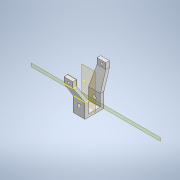
# Autodesk Inventor part: 2020_fixer2
Saved by Autodesk Inventor 2020 (Build 240168000, 168)
## iProperties
Created: 2019-10-23
Part Number: 2020_fixer2
Material: Generic
Document SubType Name: Modeling
Designer: psrob
Density: 1 g/cm^3
Appearance: Default
Author: psrob
Autodesk Inventor part; units mm, degrees
ref_plane "YZ Plane" through (0, 0, 0) normal (1, 0, 0) x (0, 1, 0)
ref_plane "XZ Plane" through (0, 0, 0) normal (0, 1, 0) x (-1, 0, 0)
ref_plane "XY Plane" through (0, 0, 0) normal (0, 0, 1) x (1, 0, 0)
sketch "Sketch1" plane through (0, 0, 0) normal (0, 0, 1) x (1, 0, 0)
  circle A0 centre (-47.5, -10) radius 3 projected
  circle A1 centre (-5, 30) radius 2 projected
  line L0 (-47.5, -10) -> (-2.5, -10)
  line L1 (7.5, 0) -> (-12.5, 0)
  line L2 (-12.5, 0) -> (-12.5, -20)
  line L3 (-12.5, -20) -> (7.5, -20)
  line L4 (7.5, -20) -> (7.5, 0)
  line L5 (7.5, 0) -> (-12.5, -20) construction
  line L6 (-12.5, 0) -> (7.5, -20) construction
  point P0 (0, 0)
  dimension "d0" = 45
  dimension "d1" = 20
  dimension "d2" = 20
  constraints: 14 end point, 2 midpoint, 2 parallel, 2 perpendicular, 1 horizontal
  measures "d0" distance of L0.start L0.end
  measures "d1" distance of L1.start L1.end
  measures "d2" distance of L2.end L1.end
extrude "Extrusion1" add sketch "Sketch1" along normal blind 6 contours L4 L3 L2 L1
ref_plane "Work Plane1" through (0, 0, -20) normal (0, 0, -1) x (-1, 0, 0)
sketch "Sketch2" plane through (0, 0, -20) normal (0, 0, -1) x (-1, 0, 0)
  line L0 (-7.5, -20) -> (-7.5, 0) projected
  line L1 (-7.5, 0) -> (12.5, 0) projected
  line L2 (12.5, 0) -> (12.5, -20) projected
  line L3 (12.5, -20) -> (-7.5, -20) projected
  point P0 (0, 0)
  dimension "d0" = 45
  dimension "d1" = 20
  dimension "d2" = 20
extrude "Extrusion2" add sketch "Sketch2" along normal blind 6
ref_plane "Work Plane2" through (-8, 25, 15) normal (0, 0, 1) x (0, 1, 0)
sketch "Sketch3" plane through (-8, 25, 15) normal (0, 0, 1) x (0, 1, 0)
  circle A0 centre (5, -3) radius 2 projected
  arc A1 (8, -10) -> (10, -8) centre (8, -8) ccw projected
  line L0 (10, -8) -> (10, -3) projected
  line L1 (10, -3) -> (10, 5) projected
  line L2 (0, 5) -> (10, 5) projected
  line L3 (0, 5) -> (0, -3) projected
  line L4 (0, -3) -> (0, -8) projected
  arc A2 (0, -8) -> (2, -10) centre (2, -8) ccw projected
  line L5 (8, -10) -> (2, -10) projected
  circle A3 centre (5, -3) radius 2 projected
  line L6 (0, 4) -> (10, 4)
  line L7 (10, 4) -> (10, -10)
  line L8 (10, -10) -> (0, -10)
  line L9 (0, -10) -> (0, 4)
  line L10 (0, 4) -> (10, -10) construction
  line L11 (10, 4) -> (0, -10) construction
  point P0 (-25, -8)
  point P1 (0, -8)
  point P2 (2, -10)
  point P3 (10, -8)
  dimension "d7" = 10
  dimension "d8" = 14
  constraints: 12 end point, 3 parallel, 2 midpoint, 1 perpendicular
  measures "d7" distance of L6.start L6.end
  measures "d8" distance of L6.end L7.end
extrude "Extrusion3" add sketch "Sketch3" along normal blind 6
sketch "Sketch4" plane through (-13, 25, 15) normal (0, -1, 0) x (1, 0, 0)
  line L0 (0, 0) -> (15, 0) projected
  line L1 (15, 0) -> (15, 6) projected
  line L2 (0, 6) -> (15, 6) projected
  line L3 (0, 0) -> (0, 6) projected
  point P0 (13, -15)
sketch "Sketch5" plane through (-12.5, 0, 0) normal (0, 1, 0) x (1, 0, 0)
  line L0 (20, 0) -> (0, 0) projected
  line L1 (0, 0) -> (0, -6) projected
  line L2 (20, -6) -> (0, -6) projected
  line L3 (20, 0) -> (20, -6) projected
  point P0 (12.5, 0)
loft "Loft1" add section 1 edges at (-2.5, 0, 0) (-12.5, 0, 3) (-2.5, 0, 6) (7.5, 0, 3) section 2 edges at (-5.5, 25, 15) (2, 25, 18) (-5.5, 25, 21) (-13, 25, 18)
ref_plane "Work Plane3" through (0, 0, -10) normal (0, 0, 1) x (1, 0, 0)
mirror "Mirror1" about plane through (0, 0, -10) normal (0, 0, 1) of "Extrusion3", "Loft1"
sketch "Sketch7" plane through (-12.5, -20, 0) normal (0, -1, 0) x (1, 0, 0)
  line L0 (0, 0) -> (20, 0) projected
  line L1 (20, 0) -> (20, 6) projected
  line L2 (0, 6) -> (20, 6) projected
  line L3 (0, 0) -> (0, 6) projected
  line L4 (20, -20) -> (0, -20) projected
  line L5 (0, -20) -> (0, -26) projected
  line L6 (20, -26) -> (0, -26) projected
  line L7 (20, -20) -> (20, -26) projected
  line L8 (20, -20) -> (20, -26) projected
  line L9 (0, 6) -> (20, 6)
  line L10 (20, 6) -> (20, -26)
  line L11 (20, -26) -> (0, -26)
  line L12 (0, -26) -> (0, 6)
  point P0 (12.5, 0)
  constraints: 8 end point, 2 parallel, 1 horizontal, 1 perpendicular
extrude "Extrusion5" add sketch "Sketch7" along normal blind 5
sketch "Sketch8" plane through (0, 0, 6) normal (0, 0, 1) x (1, 0, 0)
  line L0 (-12.5, -20) -> (7.5, -20) projected
  line L1 (-2.5, -20) -> (-2.5, -10)
  circle A0 centre (-2.5, -10) radius 3
  point P0 (0, 0)
  dimension "d23" = 10
  dimension "d24" = 6
  constraints: 2 end point, 1 centre point, 1 coincident, 1 midpoint, 1 vertical
  measures "d23" distance of L1.start L1.end
  measures "d24" diameter of A0
extrude "Extrusion6" cut sketch "Sketch8" against normal blind 40
fillet "Fillet1" radius 2 2 edges at (2, 35, 18) (2, 35, -38)
fillet "Fillet2" radius 4 2 edges at (-2.5, -25, 6) (-2.5, -25, -26)
sketch "Sketch9" plane through (-12.5, -25, 0) normal (0, -1, 0) x (1, 0, 0)
  line L0 (20, -22) -> (0, -22) projected
  line L1 (20, -22) -> (20, 2) projected
  line L2 (0, 2) -> (20, 2) projected
  line L3 (0, 2) -> (0, -22) projected
  line L4 (0, 2) -> (0, -22) projected
  line L5 (0, -22) -> (20, 2)
  line L6 (0, 2) -> (20, 2) projected
  line L7 (0, 2) -> (20, -22)
  circle A0 centre (10, -10) radius 3
  point P0 (12.5, 0)
  dimension "d29" = 6
  constraints: 4 end point, 1 centre point, 1 midpoint
  measures "d29" diameter of A0
extrude "Extrusion7" cut sketch "Sketch9" against normal blind 40 contours A0 L5 L7 | L7 L5 A0 | A0 L7 L5 | L5 L7 A0
body "Solid1"
